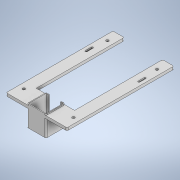
# Autodesk Inventor part: Hộp đựng động cơ
Saved by Autodesk Inventor 2020 (Build 240168000, 168)
## iProperties
Created: 2022-04-01
Part Number: Hộp đựng động cơ
Material: Generic
Document SubType Name: Modeling
Designer: PC
Density: 1 g/cm^3
Appearance: Default
Author: PC
Autodesk Inventor part; units mm, degrees
ref_plane "YZ Plane" through (0, 0, 0) normal (1, 0, 0) x (0, 1, 0)
ref_plane "XZ Plane" through (0, 0, 0) normal (0, 1, 0) x (-1, 0, 0)
ref_plane "XY Plane" through (0, 0, 0) normal (0, 0, 1) x (1, 0, 0)
sketch "Sketch1" plane through (0, 0, 0) normal (0, 1, 0) x (-1, 0, 0)
  line L0 (0, 0) -> (-47, 0)
  line L1 (-47, 0) -> (-47, -47)
  line L2 (-47, -47) -> (0, -47)
  line L3 (0, -47) -> (0, 0)
  dimension "d0" = 47
  dimension "d1" = 47
  constraints: 8 end point, 2 parallel, 1 horizontal, 1 perpendicular
  measures "d0" distance of L2.end L1.end
  measures "d1" distance of L0.end L1.end
extrude "Extrusion1" add sketch "Sketch1" along normal blind 52
sketch "Sketch2" plane through (0, 52, 0) normal (0, 1, 0) x (1, 0, 0)
  line L0 (47, 47) -> (0, 47) projected
  line L1 (47, 0) -> (47, 47) projected
  line L2 (0, 47) -> (0, 0) projected
  line L3 (0, 0) -> (47, 0) projected
  line L4 (2, 2) -> (45, 2)
  line L5 (45, 2) -> (45, 45)
  line L6 (45, 45) -> (2, 45)
  line L7 (2, 45) -> (2, 2)
  line L8 (2, 2) -> (45, 45) construction
  line L9 (45, 2) -> (2, 45) construction
  point P0 (3, 47)
  point P1 (45, 47)
  point P2 (23.5, 23.5)
  dimension "d62" = 43
  dimension "d63" = 43
  constraints: 12 end point, 2 midpoint, 2 parallel, 2 point on line, 1 horizontal, 1 perpendicular
  measures "d62" distance of L6.end L5.end
  measures "d63" distance of L5.end L4.end
extrude "Extrusion2" cut sketch "Sketch2" against normal blind 50 contours L7 L6 L5 L4
sketch "Sketch6" plane through (47, 0, 0) normal (1, 0, 0) x (0, 0, -1)
  line L0 (0, 49) -> (47, 49)
  line L1 (47, 49) -> (47, 42)
  line L2 (47, 42) -> (0, 42)
  line L3 (0, 42) -> (0, 49)
  line L4 (0, 52) -> (47, 52) projected
  dimension "d26" = 7
  dimension "d64" = 47
  dimension "d74" = 3
  constraints: 8 end point, 2 parallel, 1 horizontal, 1 perpendicular
  measures "d26" distance of L0.end L1.end
  measures "d64" distance of L1.end L2.end
  measures "d74" distance between parallel lines of L0 L4
extrude "Extrusion5" add sketch "Sketch6" along normal blind 52.5
sketch "Sketch7" plane through (47, 0, -47) normal (0, 0, -1) x (-1, 0, 0)
  line L0 (-60, 42) -> (-60, 49) projected
  line L1 (0, 42) -> (-52.5, 42) projected
  line L2 (-52.5, 49) -> (-24.5, 49)
  line L3 (-24.5, 49) -> (-24.5, 42)
  line L4 (-24.5, 42) -> (-52.5, 42)
  line L5 (-52.5, 42) -> (-52.5, 49)
  point P0 (47, 0)
  dimension "d29" = 28
  constraints: 8 end point, 2 parallel, 1 horizontal, 1 perpendicular, 1 point on line
  measures "d29" distance of L3.end L4.end
extrude "Extrusion6" add sketch "Sketch7" along normal blind 220
sketch "Sketch8" plane through (47, 49, 0) normal (0, 1, 0) x (1, 0, 0)
  line L0 (52.5, 0) -> (52.5, 267) projected
  line L1 (24.5, 267) -> (52.5, 267) projected
  line L2 (38.5, 267) -> (38.5, 0)
  line L3 (0, 0) -> (52.5, 0) projected
  circle A0 centre (38.5, 30) radius 3.25
  circle A1 centre (38.5, 238.9406) radius 3.25
  point P0 (-47, 0)
  dimension "d65" = 6.5
  dimension "d66" = 6.5
  dimension "d78" = 30
  constraints: 2 centre point, 2 end point, 2 point on line, 1 midpoint, 1 vertical
  measures "d65" diameter of A0
  measures "d66" diameter of A1
  measures "d78" distance from line of L3 A0.centre
hole "Hole1" at (85.5, 49, -30) at (85.5, 49, -238.9406) direction (0, -1, 0) diameter 4 end through all counterbore diameter 6.5 counterbore depth 4
sketch "Sketch9" plane through (47, 42, -47) normal (0, -1, 0) x (1, 0, 0)
  arc A0 (46.75, -143) -> (38.25, -143) centre (42.5, -143) ccw
  line L0 (52.5, 47) -> (52.5, -220) projected
  line L1 (0, 47) -> (52.5, 47) projected
  arc A1 (38.25, -158) -> (46.75, -158) centre (42.5, -158) ccw
  line L2 (46.75, -143) -> (46.75, -158)
  line L3 (38.25, -158) -> (38.25, -143)
  line L4 (52.5, -220) -> (24.5, -220) projected
  point P0 (-47, 47)
  dimension "d43" = 8.5
  dimension "d44" = 10
  dimension "d46" = 8.5
  dimension "d47" = 15
  dimension "d76" = 62
  constraints: 4 end point, 4 point on circle, 2 centre point, 2 tangent
  measures "d43" diameter of A0
  measures "d44" distance from line of L0 A0.centre
  measures "d46" diameter of A1
  measures "d47" distance of A1.centre A0.centre
  measures "d76" distance from line of L4 A1.centre
extrude "Extrusion7" cut sketch "Sketch9" against normal blind 4
sketch "Sketch10" plane through (47, 46, -47) normal (0, -1, 0) x (1, 0, 0)
  arc A0 (44.75, -143) -> (40.25, -143) centre (42.5, -143) ccw
  line L0 (52.5, 47) -> (52.5, -220) projected
  line L1 (0, 47) -> (52.5, 47) projected
  arc A1 (40.25, -158) -> (44.75, -158) centre (42.5, -158) ccw
  line L2 (40.25, -158) -> (40.25, -143)
  line L3 (44.75, -143) -> (44.75, -158)
  line L4 (24.5, -220) -> (52.5, -220) projected
  point P0 (-47, 47)
  dimension "d50" = 4.5
  dimension "d51" = 10
  dimension "d53" = 4.5
  dimension "d54" = 15
  dimension "d77" = 62
  constraints: 5 point on circle, 4 end point, 2 centre point, 1 parallel, 1 vertical
  measures "d50" diameter of A0
  measures "d51" distance from line of L0 A0.centre
  measures "d53" diameter of A1
  measures "d54" distance of A1.centre A0.centre
  measures "d77" distance from line of L4 A1.centre
extrude "Extrusion8" cut sketch "Sketch10" against normal blind 4
sketch "Sketch11" plane through (47, 0, -47) normal (0, 0, -1) x (-1, 0, 0)
  line L0 (0, 52) -> (47, 52) projected
  line L1 (47, 52) -> (47, 0) projected
  line L2 (2, 2) -> (45, 2) projected
  line L3 (38.5, 32) -> (38.5, 2)
  line L4 (38.5, 2) -> (8.5, 2)
  line L5 (8.5, 2) -> (8.5, 32)
  line L6 (8.5, 32) -> (38.5, 2) construction
  line L7 (38.5, 32) -> (8.5, 2) construction
  line L8 (38.5, 38) -> (38.5, 52)
  line L9 (38.5, 52) -> (8.5, 52)
  line L10 (8.5, 52) -> (8.5, 32)
  line L11 (38.5, 32) -> (38.5, 38)
  dimension "d67" = 30
  constraints: 18 end point, 2 parallel, 2 point on line, 1 vertical
  measures "d67" distance of L3.end L4.end
extrude "Extrusion9" cut sketch "Sketch11" against normal blind 2
ref_plane "Work Plane2" through (23.5, 52, -45) normal (-1, 0, 0) x (0, 0, 1)
mirror "Mirror4" about plane through (23.5, 52, -45) normal (-1, 0, 0) of "Extrusion5", "Hole1", "Extrusion6", "Extrusion8"
fillet "Fillet5" radius 3 3 edges at (-24.5, 45.5, -267) (-52.5, 45.5, -267) (-52.5, 45.5, 0)
fillet "Fillet6" radius 3 7 edges at (0, 50.5, 0) (0, 21, 0) (47, 50.5, 0) (47, 21, 0) (99.5, 45.5, -267) (71.5, 45.5, -267) (47, 21, -47)
fillet "Fillet7" radius 3 4 edges at (47, 50.5, -47) (0, 50.5, -47) (0, 21, -47) (99.5, 45.5, 0)
ref_plane "Work Plane3" through (23.5, 52, -2) normal (1, 0, 0) x (0, 0, -1)
mirror "Mirror5" about plane through (23.5, 52, -2) normal (1, 0, 0) of "Extrusion8", "Extrusion7"
body "Solid1"
